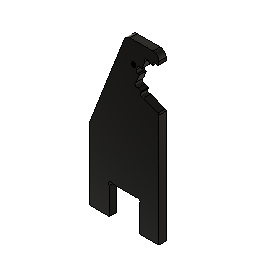
CameraTowerLeft v3 (Autodesk Fusion 360 design; units mm, degrees)
Autodesk Fusion 360 part; units mm, degrees
sketch "Sketch1" plane through (0, 0, 0) normal (0, 1, 0) x (1, 0, 0)
  line L0 (46, -110) -> (0, -110)
  line L1 (0, -110) -> (0, 0)
  line L2 (13, 0) -> (13, -17.8787)
  line L3 (15.1213, -20) -> (30.8787, -20)
  line L4 (33, -17.8787) -> (33, 0)
  line L5 (0, 0) -> (13, 0)
  line L6 (33, 0) -> (46, 0)
  line L7 (13, 0) -> (33, 0) construction
  line L8 (30.1388, -84.5498) -> (37.3876, -103.1899) construction
  line L9 (37.3876, -103.1899) -> (41.8612, -101.4502) construction
  line L10 (41.8612, -101.4502) -> (34.6124, -82.8101) construction
  line L11 (34.6124, -82.8101) -> (30.1388, -84.5498) construction
  line L12 (37.3876, -103.1899) -> (34.6124, -82.8101) construction
  line L13 (37.3876, -103.1899) -> (37.9917, -101.817) construction
  line L14 (41.8612, -101.4502) -> (40.4882, -100.8461) construction
  line L15 (30.1388, -84.5498) -> (31.5118, -85.1539) construction
  line L16 (34.6124, -82.8101) -> (34.0083, -84.183) construction
  line L17 (39.3646, -102.4211) -> (39.8841, -102.2191)
  line L18 (36.6187, -101.2128) -> (30.9076, -86.5269)
  line L19 (32.1159, -83.7809) -> (32.6354, -83.5789)
  line L20 (35.3813, -84.7872) -> (41.0924, -99.4731) construction
  arc A0 (39.3646, -102.4211) -> (36.6187, -101.2128) centre (37.9917, -101.817) ccw construction
  arc A1 (37.3876, -103.1899) -> (39.3646, -102.4211) centre (37.9917, -101.817) ccw
  arc A2 (36.6187, -101.2128) -> (37.3876, -103.1899) centre (37.9917, -101.817) ccw
  arc A3 (41.0924, -99.4731) -> (39.8841, -102.2191) centre (40.4882, -100.8461) ccw construction
  arc A4 (39.8841, -102.2191) -> (41.8612, -101.4502) centre (40.4882, -100.8461) ccw construction
  arc A5 (41.8612, -101.4502) -> (41.0924, -99.4731) centre (40.4882, -100.8461) ccw construction
  arc A6 (30.9076, -86.5269) -> (32.1159, -83.7809) centre (31.5118, -85.1539) ccw construction
  arc A7 (32.1159, -83.7809) -> (30.1388, -84.5498) centre (31.5118, -85.1539) ccw
  arc A8 (30.1388, -84.5498) -> (30.9076, -86.5269) centre (31.5118, -85.1539) ccw
  arc A9 (32.6354, -83.5789) -> (35.3813, -84.7872) centre (34.0083, -84.183) ccw construction
  arc A10 (34.6124, -82.8101) -> (32.6354, -83.5789) centre (34.0083, -84.183) ccw construction
  arc A11 (35.3813, -84.7872) -> (34.6124, -82.8101) centre (34.0083, -84.183) ccw construction
  line L21 (38.2368, -92.1301) -> (61.537, -83.0692) construction
  line L22 (57.0065, -71.4191) -> (66.0675, -94.7193) construction
  line L23 (66.0675, -94.7193) -> (44.7444, -103.0114) construction
  line L24 (57.0065, -71.4191) -> (35.6834, -79.7112) construction
  line L25 (32.6354, -83.5789) -> (34.6124, -82.8101)
  line L26 (34.6124, -82.8101) -> (34.4752, -82.4571)
  line L27 (35.6834, -79.7112) -> (46, -75.6993)
  line L28 (39.8841, -102.2191) -> (41.8612, -101.4502)
  line L29 (41.8612, -101.4502) -> (41.9984, -101.8032)
  line L30 (44.7444, -103.0114) -> (46, -102.5231)
  line L31 (46, 0) -> (46, -75.6993)
  line L32 (46, -102.5231) -> (46, -110)
  line L33 (46, -89.1112) -> (46, -102.5231) construction
  line L34 (42.7673, -103.7802) -> (43.3714, -102.4073) construction
  arc A12 (41.9984, -101.8032) -> (42.7673, -103.7802) centre (43.3714, -102.4073) ccw
  arc A13 (44.7444, -103.0114) -> (41.9984, -101.8032) centre (43.3714, -102.4073) ccw construction
  arc A14 (42.7673, -103.7802) -> (44.7444, -103.0114) centre (43.3714, -102.4073) ccw
  line L35 (41.9984, -101.8032) -> (42.7673, -103.7802) construction
  line L36 (44.7444, -103.0114) -> (42.7673, -103.7802) construction
  line L37 (42.7673, -103.7802) -> (44.7444, -103.0114) construction
  line L38 (46, -75.6993) -> (46, -89.1112) construction
  line L39 (33.7063, -80.4801) -> (35.0793, -81.0842) construction
  arc A15 (35.6834, -79.7112) -> (34.4752, -82.4571) centre (35.0793, -81.0842) ccw
  arc A16 (34.4752, -82.4571) -> (35.6834, -79.7112) centre (35.0793, -81.0842) ccw construction
  line L40 (34.4752, -82.4571) -> (33.7063, -80.4801) construction
  line L41 (35.6834, -79.7112) -> (33.7063, -80.4801) construction
  line L42 (33.7063, -80.4801) -> (35.6834, -79.7112) construction
  line L43 (36, -93) -> (29.1031, -95.682) construction
  circle A17 centre (29.1031, -95.682) radius 1.5
  line L44 (13, -20) -> (14.0607, -18.9393) construction
  line L45 (33, -20) -> (31.9393, -18.9393) construction
  arc A18 (13, -17.8787) -> (15.1213, -20) centre (14.0607, -18.9393) ccw
  arc A19 (15.1213, -20) -> (13, -17.8787) centre (14.0607, -18.9393) ccw construction
  arc A20 (30.8787, -20) -> (33, -17.8787) centre (31.9393, -18.9393) ccw
  arc A21 (33, -17.8787) -> (30.8787, -20) centre (31.9393, -18.9393) ccw construction
  line L46 (13, -17.8787) -> (13, -20) construction
  line L47 (13, -20) -> (15.1213, -20) construction
  line L48 (30.8787, -20) -> (33, -20) construction
  line L49 (33, -20) -> (33, -17.8787) construction
  line L50 (32.8571, -91.5398) -> (31.9251, -91.9023)
  line L51 (31.0707, -93.8439) -> (31.7956, -95.708)
  line L52 (33.7373, -96.5623) -> (34.6693, -96.1999)
  arc A22 (31.7956, -95.708) -> (33.7373, -96.5623) centre (33.1936, -95.1643) ccw
  arc A23 (31.9251, -91.9023) -> (31.0707, -93.8439) centre (32.4687, -93.3003) ccw
  point P0 (36, -93)
  point P1 (38.2368, -92.1301)
  point P2 (61.537, -83.0692)
  point P3 (31.4332, -94.7759)
  dimension "d2" = 110
  dimension "d3" = 20
  dimension "d4" = 20
  dimension "d5" = 13
  dimension "d6" = 46
  dimension "d7" = 13
  dimension "d15" = 20
  dimension "d16" = 4.8
  dimension "d17" = 21.25
  dimension "d18" = 1.5
  dimension "d19" = 1.5
  dimension "d20" = 45
  dimension "d21" = 45
  dimension "d22" = 1.5
  dimension "d23" = 1.5
  dimension "d24" = 45
  dimension "d25" = 45
  dimension "d26" = 25
  dimension "d29" = 84.1301
  dimension "d30" = 25.2368
  dimension "d31" = 25
  dimension "d32" = 36
  dimension "d33" = 17
  dimension "d34" = 1.5
  dimension "d35" = 45
  dimension "d36" = 1.5
  dimension "d37" = 45
  dimension "d38" = 3
  dimension "d39" = 5
  dimension "d48" = 1.5
  dimension "d49" = 1.5
  dimension "d50" = 45
  dimension "d51" = 45
  dimension "d60" = 1.5
  dimension "d61" = 1.5
  dimension "d62" = 5
  dimension "d63" = 2.5
  constraint horizontal L5
  constraint vertical L31
  constraint horizontal L0
  constraint vertical L1
  constraint coincident L1.end L5.start
  constraint perpendicular L2 L5
  constraint perpendicular L2 L3
  constraint coincident L4.end L5
  constraint perpendicular L4 L5
  constraint perpendicular L8 L9
  constraint perpendicular L9 L10
  constraint perpendicular L10 L11
  constraint midpoint L12 P0
  constraint coincident L15.end A6.centre
  constraint coincident L16.end A9.centre
  constraint coincident L13.end A0.centre
  constraint coincident L14.end A3.centre
  constraint coincident L9 L17.start
  constraint coincident L9 L17.end
  constraint coincident L8 L18.start
  constraint coincident L8 L18.end
  constraint coincident L11 L19.start
  constraint coincident L11 L19.end
  constraint coincident L10 L20.start
  constraint coincident L10 L20.end
  constraint concentric A0 A1
  constraint concentric A0 A2
  constraint concentric A3 A4
  constraint concentric A3 A5
  constraint concentric A6 A7
  constraint concentric A6 A8
  constraint concentric A9 A10
  constraint concentric A9 A11
  constraint midpoint L20 P1
  constraint coincident P1 L21.start
  constraint perpendicular L20 L21
  constraint midpoint L22 P2
  constraint coincident P2 L21.end
  constraint perpendicular L21 L22
  constraint perpendicular L22 L23
  constraint perpendicular L22 L24
  constraint perpendicular L24 L26
  constraint coincident L24 L27.end
  constraint perpendicular L23 L29
  constraint coincident L30.end L31
  constraint coincident L23 L30.end
  constraint coincident L21 L33.start
  constraint perpendicular L0 L32
  constraint coincident L34.end A12.centre
  constraint concentric A12 A13
  constraint concentric A12 A14
  constraint perpendicular L23 L35
  constraint perpendicular L22 L36
  constraint vertical L38
  constraint coincident L39.end A15.centre
  constraint coincident L39.start A15
  constraint concentric A15 A16
  constraint perpendicular L24 L40
  constraint perpendicular L22 L41
  constraint coincident P0 L43.start
  constraint perpendicular L18 L43
  constraint coincident L43.end A17.centre
  constraint coincident L44.end A18.centre
  constraint coincident L44.start A18
  constraint coincident L45.end A20.centre
  constraint coincident L45.start A20
  constraint concentric A18 A19
  constraint concentric A20 A21
  constraint perpendicular L5 L46
  constraint perpendicular L2 L47
  constraint perpendicular L2 L48
  constraint perpendicular L5 L49
  constraint coincident L8 L50.start
  constraint perpendicular L8 L50
  constraint perpendicular L50 L51
  constraint coincident L18 L52.end
  constraint perpendicular L51 L52
  constraint tangent L51 A22
  constraint tangent L52 A22
  constraint tangent L51 A23
  constraint tangent L50 A23
  constraint midpoint L51 P3
  constraint coincident L43 P3
  measures "d2" distance of L1.end L0.end
  measures "d3" distance of L2.start L44.start
  measures "d4" distance of L44.start L45.start
  measures "d5" distance of L1 L2
  measures "d6" distance of L1 L31
  measures "d7" distance of L6.end L4.end
  measures "d15" distance of L8.start L8.end
  measures "d16" distance of L8.end L9.end
  measures "d17" angle of L0 L9
  measures "d18" distance of L8.end L13.end
  measures "d19" distance of L9.end L14.end
  measures "d20" angle of L9 L13
  measures "d21" angle of L9 L14
  measures "d22" distance of L8.start L15.end
  measures "d23" distance of L10.end L16.end
  measures "d24" angle of L11 L15
  measures "d25" angle of L11 L16
  measures "d26" distance of P1 P2
  measures "d31" distance of L22.start L22.end
  measures "d32" distance of L1 P0
  measures "d33" distance of L0 P0
  measures "d34" distance of L34.start L34.end
  measures "d35" angle of L30 L34
  measures "d36" distance of L39.start L39.end
  measures "d37" angle of L24 L39
  measures "d38" diameter of A17
  measures "d39" distance of L8 L43.end
  measures "d48" distance of L44.start L44.end
  measures "d49" distance of L45.start L45.end
  measures "d50" angle of L3 L44
  measures "d51" angle of L3 L45
  measures "d60" radius of A22
  measures "d61" radius of A23
  measures "d62" distance of L50 L52
  measures "d63" distance of L8 L51
extrude "Extrude1" add sketch "Sketch1" along normal blind 4.8 contours L0 L1 L2 L3 L4 L5 L6 L17 L18 L19 A1 A2 A7 A8 L25 L26 L27 L28 L29 L30 L31 L32 A12 A14 A15 A18 A20 L50 L51 L52 A22 A23
fillet "Fillet1" radius 0.3 2 edges at (34.6124, 2.4, 82.8101) (41.8612, 2.4, 101.4502)
fillet "Fillet1" radius 1 2 edges at (46, 2.4, 102.5231) (46, 2.4, 75.6993)
fillet "Fillet1" radius 4 2 edges at (46, 2.4, 110) (0, 2.4, 110)
sketch "Sketch2" plane through (0, 0, 0) normal (0, 0, -1) x (1, 0, 0)
  line L0 (13, 0) -> (0, 0)
  line L1 (0, 0) -> (0, -4.8)
  line L2 (0, -4.8) -> (13, -4.8)
  line L3 (13, -4.8) -> (13, 0)
  line L4 (46, 0) -> (33, 0)
  line L5 (33, 0) -> (33, -4.8)
  line L6 (33, -4.8) -> (46, -4.8)
  line L7 (46, -4.8) -> (46, 0)
  line L8 (0, 0) -> (13, -4.8) construction
  line L9 (33, 0) -> (46, -4.8) construction
  circle A0 centre (6.5, -2.4) radius 1.5
  circle A1 centre (39.5, -2.4) radius 1.5
  point P0 (6.5, -2.4)
  point P1 (39.5, -2.4)
  dimension "d52" = 3
  dimension "d53" = 3
  constraint coincident L0.end L1.start
  constraint coincident L2.end L3.start
  constraint coincident L4.end L5.start
  constraint coincident L6.end L7.start
  constraint midpoint L8 P0
  constraint midpoint L9 P1
  constraint coincident P0 A0.centre
  constraint coincident P1 A1.centre
  measures "d52" diameter of A0
  measures "d53" diameter of A1
extrude "Extrude2" cut sketch "Sketch2" against normal blind 8 contours A0 | A1
thread "Thread1" "ISO Metric profile 3.0 M3x0.5 6H" major diameter 3.086 minor diameter 2.529 pitch 0.5 angle 60 modelled right hand crest width 0.1368 on face at (7.9981, 2.4748, 5.3333) crest through (7.7645, 2.4, 0.125)
thread "Thread2" "ISO Metric profile 3.0 M3x0.5 6H" major diameter 3.086 minor diameter 2.529 pitch 0.5 angle 60 modelled right hand crest width 0.1368 on face at (39.9063, 0.9561, 5.3333) crest through (40.7645, 2.4, 0.125)
thread "Thread3" "ISO Metric profile 3.0 M3x0.5 6H" major diameter 3.086 minor diameter 2.529 pitch 0.5 angle 60 modelled right hand crest width 0.1368 on face at (30.4854, 3.2, 95.0994) crest through (30.3676, 0.125, 95.682)
sketch "Sketch3" plane through (0, 0, 0) normal (0, -1, 0) x (1, 0, 0)
  arc A0 (4, 110) -> (0, 106) centre (4, 106) ccw
  line L0 (0, 106) -> (0, 0)
  line L1 (0, 0) -> (13, 0)
  line L2 (13, 0) -> (13, 17.8787)
  arc A1 (15.1213, 20) -> (13, 17.8787) centre (14.0607, 18.9393) ccw
  line L3 (15.1213, 20) -> (30.8787, 20)
  arc A2 (33, 17.8787) -> (30.8787, 20) centre (31.9393, 18.9393) ccw
  line L4 (33, 17.8787) -> (33, 0)
  line L5 (33, 0) -> (46, 0)
  line L6 (46, 0) -> (46, 75.0152)
  arc A3 (46, 75.0152) -> (45.3624, 75.9472) centre (45, 75.0152) ccw
  line L7 (45.3624, 75.9472) -> (35.6834, 79.7112)
  arc A4 (34.4752, 82.4571) -> (35.6834, 79.7112) centre (35.0793, 81.0842) ccw
  line L8 (34.4752, 82.4571) -> (34.5037, 82.5305)
  arc A5 (34.5037, 82.5305) -> (34.3328, 82.9188) centre (34.2241, 82.6392) ccw
  line L9 (34.3328, 82.9188) -> (32.1159, 83.7809)
  arc A6 (30.9076, 86.5269) -> (32.1159, 83.7809) centre (31.5118, 85.1539) ccw
  line L10 (30.9076, 86.5269) -> (32.8571, 91.5398)
  arc A7 (39.3646, 102.4211) -> (36.6187, 101.2128) centre (37.9917, 101.817) ccw
  line L11 (39.3646, 102.4211) -> (41.5816, 101.559)
  arc A8 (41.5816, 101.559) -> (41.9699, 101.7298) centre (41.6903, 101.8386) ccw
  line L12 (41.9699, 101.7298) -> (41.9984, 101.8032)
  arc A9 (44.7444, 103.0114) -> (41.9984, 101.8032) centre (43.3714, 102.4073) ccw
  arc A10 (44.7444, 103.0114) -> (46, 103.9782) centre (45, 103.9782) ccw
  line L13 (46, 103.9782) -> (46, 106)
  arc A11 (46, 106) -> (42, 110) centre (42, 106) ccw
  line L14 (42, 110) -> (4, 110)
  spline S0 degree 3 poles (30.0613, 96.5073) (30.1833, 96.3932) (30.2815, 96.2561) (30.4238, 95.946) (30.4642, 95.775) (30.4788, 95.4202) (30.4502, 95.2398) (30.3243, 94.8929) (30.2258, 94.7308) (30.0187, 94.5029) (29.9276, 94.4243) (29.7264, 94.2891) (29.6167, 94.2334) (29.5017, 94.1914) knots 0 0 0 0 0.050111 0.050111 0.102261 0.102261 0.15645 0.15645 0.212677 0.212677 0.24852 0.24852 0.285143 0.285143 0.285143 0.285143
  arc A12 (28.7046, 94.1914) -> (29.5017, 94.1914) centre (29.1031, 95.682) ccw
  spline S1 degree 3 poles (28.7046, 94.1914) (28.5198, 94.2589) (28.3497, 94.3613) (28.0642, 94.6219) (27.9499, 94.7756) (27.7907, 95.1125) (27.7451, 95.2912) (27.7265, 95.6494) (27.7511, 95.8252) (27.8442, 96.0902) (27.8906, 96.1848) (28.0041, 96.3585) (28.0702, 96.4373) (28.145, 96.5073) knots 0 0 0 0 0.059039 0.059039 0.116033 0.116033 0.170983 0.170983 0.223888 0.223888 0.255505 0.255505 0.286347 0.286347 0.286347 0.286347
  arc A13 (30.0613, 96.5073) -> (28.145, 96.5073) centre (29.1031, 95.682) ccw
  line L15 (23.9416, 110) -> (0, 48.4344)
  line L16 (30.1388, 84.5498) -> (37.3876, 103.1899)
  line L17 (36.6187, 101.2128) -> (30.9076, 86.5269)
  line L18 (32.8571, 91.5398) -> (31.9251, 91.9023)
  arc A14 (31.0707, 93.8439) -> (31.9251, 91.9023) centre (32.4687, 93.3003) ccw
  line L19 (31.0707, 93.8439) -> (31.7956, 95.708)
  arc A15 (33.7373, 96.5623) -> (31.7956, 95.708) centre (33.1936, 95.1643) ccw
  line L20 (33.7373, 96.5623) -> (34.6693, 96.1999)
  line L21 (34.6693, 96.1999) -> (36.6187, 101.2128)
  dimension "d56" = 15
  constraint coincident L14 L15.start
  constraint coincident L0 L15.end
  constraint parallel L15 L16
  measures "d56" distance of L15 L17
extrude "Extrude3" cut sketch "Sketch3" against normal through all contours A0 L0 L14 L15
fillet "Fillet2" radius 4 2 edges at (23.9416, 2.4, 110) (0, 2.4, 48.4344)
